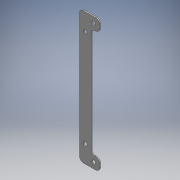
# Autodesk Inventor part: side
Saved by Autodesk Inventor 2016 (Build 200138000, 138)
## iProperties
Created: 2022-06-29
Part Number: side
Material: Generic
Document SubType Name: Modeling
Designer: Teemu S.
Density: 1 g/cm^3
Appearance: Default
Author: Teemu S.
Autodesk Inventor part; units mm, degrees
ref_plane "YZ Plane" through (0, 0, 0) normal (1, 0, 0) x (0, 1, 0)
ref_plane "XZ Plane" through (0, 0, 0) normal (0, 1, 0) x (-1, 0, 0)
ref_plane "XY Plane" through (0, 0, 0) normal (0, 0, 1) x (1, 0, 0)
sketch "Sketch1" plane through (0, 0, 0) normal (0, 1, 0) x (-1, 0, 0)
  line L0 (0, 0) -> (144.5, 0) construction
  line L1 (144.5, 0) -> (144.5, -204.5) construction
  line L2 (144.5, -204.5) -> (0, -204.5) construction
  line L3 (0, -204.5) -> (0, 0) construction
  circle A0 centre (135.5, -27) radius 3 construction
  circle A1 centre (122.5, -9) radius 3 construction
  circle A2 centre (135.5, -177.5) radius 3 construction
  circle A3 centre (122.5, -195.5) radius 3 construction
  circle A4 centre (22, -195.5) radius 3 construction
  circle A5 centre (9, -177.5) radius 3 construction
  circle A6 centre (9, -27) radius 3 construction
  circle A7 centre (22, -9) radius 3 construction
  line L4 (12, -12) -> (132.5, -12) construction
  line L5 (132.5, -12) -> (132.5, -192.5) construction
  line L6 (132.5, -192.5) -> (12, -192.5) construction
  line L7 (12, -192.5) -> (12, -12) construction
  circle A8 centre (22, -9) radius 2.925
  circle A9 centre (9, -27) radius 2.925
  circle A10 centre (122.5, -9) radius 2.925
  circle A11 centre (135.5, -27) radius 2.925
  circle A12 centre (135.5, -177.5) radius 2.925
  circle A13 centre (122.5, -195.5) radius 2.925
  circle A14 centre (22, -195.5) radius 2.925
  circle A15 centre (9, -177.5) radius 2.925
  line L8 (122.5, -9) -> (135.5, -9) construction
  line L9 (135.5, -9) -> (135.5, -27) construction
  line L10 (126.5, -27) -> (126.5, -18)
  line L11 (126.5, -18) -> (122.5, -18)
  line L12 (144.5, -27) -> (144.5, 0)
  line L13 (144.5, 0) -> (122.5, 0)
  line L14 (122.5, -195.5) -> (135.5, -195.5) construction
  line L15 (135.5, -195.5) -> (135.5, -177.5) construction
  line L16 (126.5, -177.5) -> (126.5, -186.5)
  line L17 (126.5, -186.5) -> (122.5, -186.5)
  line L18 (144.5, -177.5) -> (144.5, -204.5)
  line L19 (144.5, -204.5) -> (122.5, -204.5)
  line L20 (126.5, -27) -> (126.5, -177.5)
  line L21 (144.5, -177.5) -> (144.5, -27)
  line L22 (122.5, -9) -> (113.5, -9) construction
  line L23 (122.5, 0) -> (113.5, 0)
  line L24 (122.5, -18) -> (113.5, -18)
  line L25 (113.5, -18) -> (113.5, 0)
  line L26 (122.5, -195.5) -> (113.5, -195.5) construction
  line L27 (122.5, -204.5) -> (113.5, -204.5)
  line L28 (122.5, -186.5) -> (113.5, -186.5)
  line L29 (113.5, -186.5) -> (113.5, -204.5)
  line L30 (75.275, -87.25) -> (69.225, -87.25) construction
  line L31 (69.225, -87.25) -> (69.225, -117.25) construction
  line L32 (69.225, -117.25) -> (75.275, -117.25) construction
  line L33 (75.275, -117.25) -> (75.275, -87.25) construction
  line L34 (75.185, -87.75) -> (73.8621, -87.75)
  line L35 (69.315, -87.75) -> (69.315, -91.25)
  line L36 (69.315, -116.75) -> (70.6379, -116.75)
  line L37 (75.185, -116.75) -> (75.185, -113.25)
  arc A16 (73.8621, -116.75) -> (75.185, -113.25) centre (75.185, -115.25) ccw
  arc A17 (69.315, -113.25) -> (70.6379, -116.75) centre (69.315, -115.25) ccw
  arc A18 (75.185, -91.25) -> (73.8621, -87.75) centre (75.185, -89.25) ccw
  arc A19 (70.6379, -87.75) -> (69.315, -91.25) centre (69.315, -89.25) ccw
  line L38 (69.315, -91.25) -> (69.315, -113.25)
  line L39 (70.6379, -87.75) -> (69.315, -87.75)
  line L40 (73.8621, -87.75) -> (70.6379, -87.75)
  line L41 (75.185, -91.25) -> (75.185, -87.75)
  line L42 (75.185, -113.25) -> (75.185, -91.25)
  line L43 (70.6379, -116.75) -> (73.8621, -116.75)
  line L44 (73.8621, -116.75) -> (75.185, -116.75)
  line L45 (69.315, -113.25) -> (69.315, -116.75)
  arc A20 (69.315, -91.25) -> (70.6379, -87.75) centre (69.315, -89.25) ccw
  arc A21 (73.8621, -87.75) -> (75.185, -91.25) centre (75.185, -89.25) ccw
  arc A22 (75.185, -113.25) -> (73.8621, -116.75) centre (75.185, -115.25) ccw
  arc A23 (70.6379, -116.75) -> (69.315, -113.25) centre (69.315, -115.25) ccw
  point P0 (132.5, -102.25)
  point P1 (144.5, -102.25)
  point P2 (72.25, -12)
  point P3 (72.25, 0)
  point P4 (72.25, -87.25)
  point P5 (75.275, -102.25)
  point P6 (75.185, -102.25)
  point P7 (72.25, -87.75)
  point P8 (75.185, -102.25)
  point P9 (72.25, -87.75)
  dimension "d0" = 144.5
  dimension "d1" = 204.5
  dimension "d2" = 6
  dimension "d3" = 6
  dimension "d4" = 6
  dimension "d5" = 6
  dimension "d6" = 6
  dimension "d7" = 6
  dimension "d8" = 6
  dimension "d9" = 6
  dimension "d10" = 120.5
  dimension "d11" = 180.5
  dimension "d12" = 15
  dimension "d13" = 10
  dimension "d14" = 10
  dimension "d15" = 15
  dimension "d16" = 15
  dimension "d17" = 10
  dimension "d18" = 10
  dimension "d19" = 15
  dimension "d20" = 0.075
  dimension "d21" = 0.075
  dimension "d22" = 0.075
  dimension "d23" = 0.075
  dimension "d24" = 0.075
  dimension "d25" = 0.075
  dimension "d26" = 0.075
  dimension "d27" = 0.075
  dimension "d28" = 9
  dimension "d29" = 9
  dimension "d30" = 9
  dimension "d31" = 9
  dimension "d32" = 9
  dimension "d33" = 9
  dimension "pcbH" = 6.05
  dimension "pcbW" = 30
  dimension "pcbWcut" = 29
  dimension "pcbHcut" = 5.87
  dimension "clearance" = 4
  dimension "d42" = 1.5
  dimension "d43" = 4
  dimension "d44" = 1.5
  dimension "d45" = 1.5
  dimension "d46" = 1.5
  dimension "d47" = 4
  dimension "d48" = 4
  constraints: 92 end point, 24 centre point, 24 parallel, 20 perpendicular, 16 point on circle, 12 horizontal, 10 midpoint, 9 point on line, 8 coincident, 8 tangent, 4 horizontal alignment, 4 vertical alignment, 4 other
  measures "d0" distance of L1.end L2.end
  measures "d1" distance of L0.end L1.end
  measures "d2" diameter of A0
  measures "d3" diameter of A1
  measures "d4" diameter of A2
  measures "d5" diameter of A3
  measures "d6" diameter of A4
  measures "d7" diameter of A5
  measures "d8" diameter of A6
  measures "d9" diameter of A7
  measures "d10" distance of L5.end L6.end
  measures "d11" distance of L4.end L5.end
  measures "d12" vertical distance of A0.centre L4.end
  measures "d13" horizontal distance of L4.end A1.centre
  measures "d14" horizontal distance of L4.start A7.centre
  measures "d15" vertical distance of L4.start A6.centre
  measures "d16" vertical distance of L6.end A5.centre
  measures "d17" horizontal distance of A4.centre L6.end
  measures "d18" horizontal distance of L5.end A3.centre
  measures "d19" vertical distance of L5.end A2.centre
  measures "d20" radial gap between concentric circles of A5 A15
  measures "d21" radial gap between concentric circles of A4 A14
  measures "d22" radial gap between concentric circles of A6 A9
  measures "d23" radial gap between concentric circles of A7 A8
  measures "d24" radial gap between concentric circles of A1 A10
  measures "d25" radial gap between concentric circles of A0 A11
  measures "d26" radial gap between concentric circles of A2 A12
  measures "d27" radial gap between concentric circles of A3 A13
  measures "d28" distance between parallel lines of L9 L10
  measures "d29" distance between parallel lines of L9 L12
  measures "d30" distance between parallel lines of L15 L16
  measures "d31" distance between parallel lines of L15 L18
  measures "d32" distance of L8.start L22.end
  measures "d33" distance of L14.start L26.end
  measures "pcbH" distance of L32.end L31.end
  measures "pcbW" distance of L30.end L31.end
  measures "pcbWcut" distance of L37.start L34.start
  measures "pcbHcut" distance of L34.start L35.start
  measures "clearance" diameter of A16
  measures "d42" distance of A16.centre L37.start
  measures "d43" diameter of A17
  measures "d44" distance of L36.start A17.centre
  measures "d45" distance of L34.start A18.centre
  measures "d46" distance of L35.start A19.centre
  measures "d47" diameter of A18
  measures "d48" diameter of A19
extrude "Extrusion1" add sketch "Sketch1" along normal blind 1.5 contours L10 L11 L24 L25 L23 L13 L12 L21 L18 L19 L27 L29 L28 L17 L16 L20
fillet "Fillet1" radius 6 8 edges at (-144.5, 0.75, 0) (-113.5, 0.75, 0) (-113.5, 0.75, -18) (-126.5, 0.75, -18) (-126.5, 0.75, -186.5) (-113.5, 0.75, -186.5) (-113.5, 0.75, -204.5) (-144.5, 0.75, -204.5)
equation "\"d0\" = height"
equation "\"d1\" = width"
equation "\"d2\" = pinD"
equation "\"d3\" = pinD"
equation "\"d4\" = pinD"
equation "\"d5\" = pinD"
equation "\"d6\" = pinD"
equation "\"d7\" = pinD"
equation "\"d8\" = pinD"
equation "\"d9\" = pinD"
equation "\"d10\" = stencilH"
equation "\"d11\" = stencilW"
equation "\"d12\" = cornerW"
equation "\"d13\" = cornerH"
equation "\"d14\" = cornerH"
equation "\"d15\" = cornerW"
equation "\"d16\" = cornerW"
equation "\"d17\" = cornerH"
equation "\"d18\" = cornerH"
equation "\"d19\" = cornerW"
equation "\"d20\" = kerf"
equation "\"d21\" = kerf"
equation "\"d22\" = kerf"
equation "\"d23\" = kerf"
equation "\"d24\" = kerf"
equation "\"d25\" = kerf"
equation "\"d26\" = kerf"
equation "\"d27\" = kerf"
equation "\"d28\" = 1.5 * pinD"
equation "\"d29\" = 1.5 * pinD"
equation "\"d30\" = 1.5 * pinD"
equation "\"d31\" = 1.5 * pinD"
equation "\"d32\" = 1.5 * pinD"
equation "\"d33\" = 1.5 * pinD"
equation "\"d43\" = clearance"
equation "\"d44\" = d42"
equation "\"d45\" = d42"
equation "\"d46\" = d45"
equation "\"d47\" = clearance"
equation "\"d48\" = clearance"
equation "\"d36\" = pinD"
equation "\"height\" = 144.5"
equation "\"width\" = 204.5"
equation "\"pinD\" = 6"
equation "\"stencilH\" = 120.5"
equation "\"stencilW\" = 180.5"
equation "\"cornerW\" = 15"
equation "\"cornerH\" = 10"
equation "\"kerf\" = 0.075"
body "Solid1"
